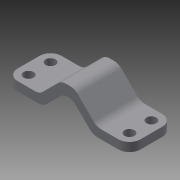
# Autodesk Inventor part: clip_cover
Saved by Autodesk Inventor 2013 (Build 170138000, 138)
## iProperties
Created: 2013-03-18
Part Number: clip_cover
Material: Generic
Document SubType Name: Modeling
Designer: Mahisorn
Density: 1 g/cm^3
Author: Mahisorn
Autodesk Inventor part; units mm, degrees
ref_plane "YZ Plane" through (0, 0, 0) normal (1, 0, 0) x (0, 1, 0)
ref_plane "XZ Plane" through (0, 0, 0) normal (0, 1, 0) x (-1, 0, 0)
ref_plane "XY Plane" through (0, 0, 0) normal (0, 0, 1) x (1, 0, 0)
sketch "Sketch1" plane through (0, 0, 0) normal (0, 1, 0) x (-1, 0, 0)
  line L0 (-3, 0) -> (-13, -10)
  line L1 (-13, -10) -> (-28, -10)
  line L2 (-28, -14) -> (-11.3431, -14)
  line L3 (-11.3431, -14) -> (0, -2.6569)
  line L4 (-28, -10) -> (-28, -14)
  line L5 (-3, 0) -> (0, 0)
  line L6 (0, 0) -> (0, -2.6569)
  dimension "d7" = 15
  dimension "d9" = 4
  dimension "d38" = 10
  dimension "d39" = 4
  constraints: 14 end point, 3 perpendicular, 1 parallel
  measures "d7" distance of L0.end L1.end
  measures "d9" distance between parallel lines of L3 L0
  measures "d38" horizontal distance of L0.end L0.start
  measures "d39" distance of L1.end L2.start
extrude "Extrusion1" add sketch "Sketch1" along normal blind 20
sketch "Sketch4" plane through (13, 0, -10) normal (0, 0, 1) x (1, 0, 0)
  line L0 (0, 20) -> (15, 20) projected
  line L1 (15, 0) -> (15, 20) projected
  point P0 (-13, 0)
  point P1 (10, 15)
  point P2 (10, 5)
  dimension "d28" = 5
  dimension "d29" = 10
  dimension "d40" = 5
  constraints: 1 vertical alignment
  measures "d28" distance from line of point (10, 15) L0
  measures "d29" distance of point (10, 5) point (10, 15)
  measures "d40" distance from line of L1 point (10, 15)
hole "Hole3" at (23, 15, -10) at (23, 5, -10) direction (0, 0, -1) diameter 4.5 end through all clearance for "Flat Head Machine Screw" size "M4" standard "Ansi Metric M Profile"
fillet "Fillet4" radius 5 5 edges at (28, 20, -12) (28, 0, -12) (11.3431, 10, -14) (13, 10, -10) (3, 10, 0)
mirror "Mirror3" about plane through (0, 0, -2.6569) normal (-1, 0, 0) of "Extrusion1", "Fillet4", "Hole3"
fillet "Fillet5" radius 5 1 edges at (0, 10, -2.6569)
body "Solid1"
